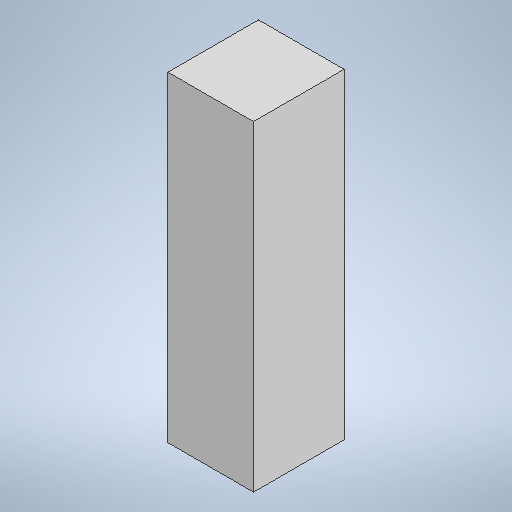
# Autodesk Inventor part: EndCap
Saved by Autodesk Inventor 2025.2 (Build 292293000, 293)
## iProperties
Created: 2025-03-30
Part Number: EndCap
Material: Generic
Document SubType Name: Modeling
Designer: georg
Density: 1 g/cm^3
Appearance: Default
Author: georg
Autodesk Inventor part; units mm, degrees
ref_plane "YZ Plane" through (0, 0, 0) normal (1, 0, 0) x (0, 1, 0)
ref_plane "XZ Plane" through (0, 0, 0) normal (0, 1, 0) x (-1, 0, 0)
ref_plane "XY Plane" through (0, 0, 0) normal (0, 0, 1) x (1, 0, 0)
sketch "Sketch1" plane through (0, 0, 0) normal (0, 0, 1) x (1, 0, 0)
  line L0 (6, -22.5) -> (-6, -22.5)
  line L1 (-6, -22.5) -> (-6, 22.5)
  line L2 (-6, 22.5) -> (6, 22.5)
  line L3 (6, 22.5) -> (6, -22.5)
  line L4 (6, -22.5) -> (-6, 22.5) construction
  line L5 (-6, -22.5) -> (6, 22.5) construction
  line L6 (-5.1503, -35.0501) -> (13.5409, -35.0501)
  point P0 (0, 0)
  point P1 (4.1953, 105.9109)
  point P2 (0, 0)
  point P3 (11.236, -97.2891)
  point P4 (-6, 0)
  dimension "d0" = 12
  dimension "d1" = 45
  dimension "d2" = 57.55
  constraints: 12 end point, 3 midpoint, 2 parallel, 1 coincident, 1 horizontal, 1 perpendicular, 3 other
  measures "d0" distance between parallel lines of L3 L1
  measures "d1" distance of L2.end L0.start
extrude "Extrusion1" add sketch "Sketch1" along normal blind 12.7
sketch "Sketch3" plane through (-6, -22.5, 0) normal (-1, 0, 0) x (0, 0, 1)
  circle A0 centre (6.35, 38.65) radius 3.175
  line L0 (12.7, 45) -> (12.7, 0) projected
  line L1 (0, 45) -> (12.7, 45) projected
  circle A1 centre (6.35, 6.35) radius 3.175
  line L2 (0, 0) -> (12.7, 0) projected
  point P0 (0, 22.5)
  point P1 (6.35, 45)
  dimension "d10" = 6.35
  dimension "d11" = 6.35
  dimension "d12" = 6.35
  dimension "d13" = 6.35
  dimension "d14" = 6.35
  dimension "d15" = 6.35
  constraints: 2 centre point, 1 midpoint
  measures "d10" diameter of A0
  measures "d11" distance from line of L0 A0.centre
  measures "d12" distance of point (6.35, 45) A0.centre
  measures "d13" diameter of A1
  measures "d14" distance from line of L2 A1.centre
  measures "d15" distance from line of L0 A1.centre
extrude "Extrusion3" cut sketch "Sketch3" against normal blind 6.35
body "Solid1"
